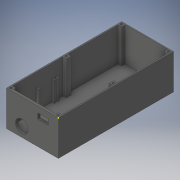
# Autodesk Inventor part: Housing Rev 3
Saved by Autodesk Inventor 2018 (Build 220112000, 112)
## iProperties
Created: 2018-02-03
Part Number: Housing Rev 3
Material: Generic
Document SubType Name: Modeling
Designer: Mom
Density: 1 g/cm^3
Appearance: Default
Author: Mom
Autodesk Inventor part; units mm, degrees
ref_plane "YZ Plane" through (0, 0, 0) normal (1, 0, 0) x (0, 1, 0)
ref_plane "XZ Plane" through (0, 0, 0) normal (0, 1, 0) x (-1, 0, 0)
ref_plane "XY Plane" through (0, 0, 0) normal (0, 0, 1) x (1, 0, 0)
sketch "Sketch2" plane through (0, 0, 0) normal (0, 1, 0) x (-1, 0, 0)
  line L0 (0, 0) -> (0, -200)
  line L1 (0, -200) -> (90, -200)
  line L2 (90, -200) -> (90, 0)
  line L3 (90, 0) -> (0, 0)
  line L4 (0, 0) -> (0, -8)
  line L5 (2, -96) -> (8, -96)
  line L6 (8, -96) -> (8, -104)
  line L7 (8, -104) -> (2, -104)
  line L8 (2, -104) -> (2, -192)
  line L9 (2, -192) -> (8, -192)
  line L10 (8, -192) -> (8, -198)
  line L11 (8, -198) -> (45, -198)
  line L12 (8, -4) -> (45, -4)
  line L13 (8, -4) -> (8, -8)
  line L14 (88, -96) -> (82, -96)
  line L15 (82, -96) -> (82, -104)
  line L16 (82, -104) -> (88, -104)
  line L17 (88, -104) -> (88, -192)
  line L18 (88, -192) -> (82, -192)
  line L19 (82, -192) -> (82, -198)
  line L20 (82, -198) -> (45, -198)
  line L21 (82, -4) -> (45, -4)
  line L22 (82, -4) -> (82, -8)
  line L23 (90, -200) -> (90, -196)
  line L24 (0, -200) -> (0, -196)
  circle A0 centre (4, -196) radius 2.1
  circle A1 centre (86, -196) radius 2.1
  circle A2 centre (86, -100) radius 2.1
  circle A3 centre (86, -4) radius 2.1
  circle A4 centre (4, -4) radius 2.1
  circle A5 centre (4, -100) radius 2.1
  line L25 (6, -86) -> (6, -83)
  line L26 (6, -86) -> (2, -86)
  line L27 (2, -86) -> (2, -96)
  line L28 (6, -83) -> (2, -83)
  line L29 (2, -83) -> (2, -80)
  line L30 (2, -80) -> (6, -80)
  line L31 (6, -80) -> (6, -77)
  line L32 (6, -77) -> (2, -77)
  line L33 (84, -86) -> (84, -83)
  line L34 (84, -86) -> (88, -86)
  line L35 (84, -83) -> (88, -83)
  line L36 (88, -83) -> (88, -80)
  line L37 (88, -80) -> (84, -80)
  line L38 (84, -80) -> (84, -77)
  line L39 (84, -77) -> (88, -77)
  line L40 (88, -86) -> (88, -96)
  line L41 (84, -8) -> (84, -11)
  line L42 (84, -11) -> (88, -11)
  line L43 (88, -50) -> (84, -50)
  line L44 (84, -50) -> (84, -53)
  line L45 (84, -53) -> (88, -53)
  line L46 (82, -8) -> (84, -8)
  line L47 (88, -11) -> (88, -50)
  line L48 (88, -53) -> (88, -77)
  line L49 (6, -8) -> (6, -11)
  line L50 (6, -11) -> (2, -11)
  line L51 (2, -50) -> (6, -50)
  line L52 (6, -50) -> (6, -53)
  line L53 (6, -53) -> (2, -53)
  line L54 (8, -8) -> (6, -8)
  line L55 (2, -11) -> (2, -50)
  line L56 (2, -53) -> (2, -77)
  dimension "d1" = 200
  dimension "d2" = 90
  dimension "d3" = 200
  dimension "d4" = 8
  dimension "d5" = 8
  dimension "d8" = 6
  dimension "d9" = 8
  dimension "d10" = 6
  dimension "d11" = 88
  dimension "d12" = 6
  dimension "d13" = 6
  dimension "d41" = 4
  dimension "d43" = 4
  dimension "d45" = 4.2
  dimension "d46" = 4.2
  dimension "d47" = 4.2
  dimension "d48" = 4.2
  dimension "d49" = 4.2
  dimension "d50" = 4.2
  dimension "d87" = 3
  dimension "d88" = 4
  dimension "d89" = 4
  dimension "d90" = 3
  dimension "d92" = 4
  dimension "d93" = 3
  dimension "d94" = 4
  dimension "d96" = 3
  dimension "d98" = 3
  constraints: 114 end point, 8 perpendicular, 7 point on line, 6 centre point, 4 vertical, 3 horizontal, 3 parallel
  measures "d1" distance of L0.start L0.end
  measures "d2" distance of L0.end L1.end
  measures "d3" distance of L1.end L2.end
  measures "d4" distance of L0.start L4.end
  measures "d5" distance of L4.end L13.end
  measures "d8" distance of L5.start L5.end
  measures "d9" distance of L5.end L6.end
  measures "d10" distance of L6.end L7.end
  measures "d11" distance of L7.end L8.end
  measures "d12" distance of L8.end L9.end
  measures "d13" distance of L9.end L10.end
  measures "d41" distance of L1.end L23.end
  measures "d43" distance of L0.end L24.end
  measures "d45" diameter of A0
  measures "d46" diameter of A1
  measures "d47" diameter of A2
  measures "d48" diameter of A3
  measures "d49" diameter of A4
  measures "d50" diameter of A5
  measures "d87" distance of L25.start L25.end
  measures "d88" distance of L25.start L26.end
  measures "d89" distance of L25.end L28.end
  measures "d90" distance of L28.end L29.end
  measures "d92" distance of L29.end L30.end
  measures "d93" distance of L30.end L31.end
  measures "d94" distance of L31.end L32.end
  measures "d96" distance of L41.start L41.end
  measures "d98" distance of L43.end L44.end
extrude "Extrusion1" add sketch "Sketch2" along normal blind 59
sketch "Sketch11" plane through (-90, 0, 0) normal (0, 0, 1) x (1, 0, 0)
  circle A0 centre (26.5144, 14.75) radius 11
  line L0 (63.5431, 48.75) -> (72.5431, 48.75)
  line L1 (72.5431, 48.75) -> (72.5431, 39.75)
  line L2 (72.5431, 39.75) -> (54.5431, 39.75)
  line L3 (54.5431, 39.75) -> (54.5431, 48.75)
  line L4 (54.5431, 48.75) -> (63.5431, 48.75)
  dimension "d76" = 22
  dimension "d78" = 9
  dimension "d79" = 9
  dimension "d80" = 18
  dimension "d81" = 9
  constraints: 10 end point, 2 perpendicular, 1 centre point, 1 point on line
  measures "d76" diameter of A0
  measures "d78" distance of L0.start L0.end
  measures "d79" distance of L0.end L1.end
  measures "d80" distance of L1.end L2.end
  measures "d81" distance of L2.end L3.end
extrude "Extrusion7" cut sketch "Sketch11" against normal blind 5
sketch "Sketch12" plane through (0, 59, 0) normal (0, 1, 0) x (1, 0, 0)
  point P0 (0, 0)
sketch "Sketch13" plane through (-84, 0, -86) normal (0, 0, -1) x (-1, 0, 0)
  line L0 (0, 35) -> (4, 35)
  line L1 (0, 35) -> (0, 59)
  line L2 (0, 59) -> (4, 59) projected
  line L3 (0, 59) -> (4, 59)
  line L4 (4, 59) -> (4, 35)
  point P0 (-84, 0)
  point P1 (4, 0)
  point P2 (0, 0)
  constraints: 8 end point, 1 collinear
extrude "Extrusion8" cut sketch "Sketch13" against normal blind 78
sketch "Sketch14" plane through (-2, 0, -86) normal (0, 0, -1) x (-1, 0, 0)
  line L0 (4, 0) -> (4, 59) projected
  line L1 (4, 0) -> (4, 35)
  line L2 (4, 0) -> (39, 0) construction
  line L3 (4, 35) -> (0, 35)
  line L4 (0, 0) -> (0, 59) projected
  line L5 (0, 35) -> (0, 59)
  line L6 (0, 59) -> (4, 59)
  line L7 (4, 59) -> (4, 35)
  point P0 (-2, 0)
  dimension "d104" = 35
  dimension "d105" = 90
  constraints: 12 end point, 4 perpendicular, 2 collinear, 1 horizontal, 1 point on line
  measures "d104" distance of L0.start L1.end
  measures "d105" angle of L2 L1
extrude "Extrusion9" cut sketch "Sketch14" against normal blind 78
sketch "Sketch15" plane through (0, 0, 0) normal (0, -1, 0) x (1, 0, 0)
  line L0 (-90, 0) -> (0, 0) projected
  line L1 (0, -200) -> (-90, -200) projected
  line L2 (0, 0) -> (0, -200)
  line L3 (0, -200) -> (-90, -200)
  line L4 (-90, -200) -> (-90, 0)
  line L5 (-90, 0) -> (0, 0)
  constraints: 8 end point, 3 perpendicular, 1 vertical
extrude "Extrusion10" add sketch "Sketch15" along normal blind 2
body "Solid1"
